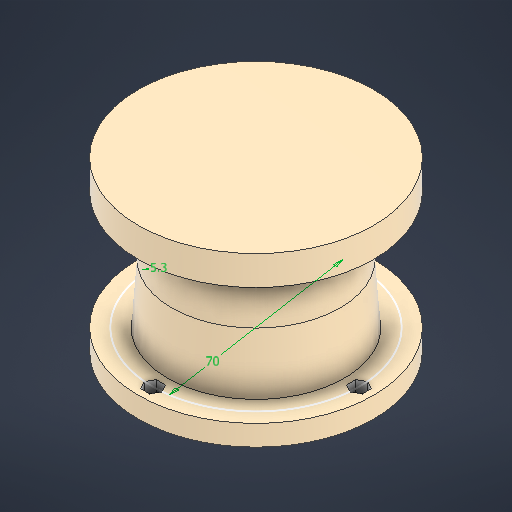
# Autodesk Inventor part: spool
Saved by Autodesk Inventor 2026.2 (Build 302298010, 298A)
## iProperties
Created: 2026-02-24
Part Number: spool
Material: ABS Plastic
Document SubType Name: Modeling
Designer: Luke
Density: 1.06 g/cm^3
Appearance: Smooth - White
Author: Luke
Autodesk Inventor part; units mm, degrees
ref_plane "YZ Plane" through (0, 0, 0) normal (1, 0, 0) x (0, 1, 0)
ref_plane "XZ Plane" through (0, 0, 0) normal (0, 1, 0) x (-1, 0, 0)
ref_plane "XY Plane" through (0, 0, 0) normal (0, 0, 1) x (1, 0, 0)
sketch "Sketch1" plane through (0, 0, 0) normal (0, 1, 0) x (-1, 0, 0)
  circle A0 centre (0, 0) radius 30
  circle A1 centre (0, 0) radius 45
  circle A2 centre (0, 0) radius 20
  dimension "d0" = 60
  dimension "d1" = 90
  dimension "d2" = 40
  constraints: 3 centre point, 3 coincident
  measures "d0" diameter of A0
  measures "d1" diameter of A1
  measures "d2" diameter of A2
extrude "Extrusion1" add sketch "Sketch1" along normal blind 20 draft -4 contours A0
sketch "Sketch2" plane through (0, 20, 0) normal (0, 1, 0) x (1, 0, 0)
  circle A0 centre (0, 0) radius 28.6015
  circle A1 centre (0, 0) radius 21.3985
  constraints: 2 centre point, 2 coincident
extrude "Extrusion2" add sketch "Sketch2" along normal blind 20 draft 4
sketch "Sketch3" plane through (0, 40, 0) normal (0, 1, 0) x (1, 0, 0)
  circle A0 centre (0, 0) radius 40
  dimension "d7" = 80
  constraints: 1 centre point, 1 coincident
  measures "d7" diameter of A0
extrude "Extrusion3" add sketch "Sketch3" along normal blind 10
sketch "Sketch4" plane through (0, 0, 0) normal (0, -1, 0) x (1, 0, 0)
  circle A0 centre (0, 0) radius 40
  dimension "d10" = 80
  constraints: 1 centre point, 1 coincident
  measures "d10" diameter of A0
extrude "Extrusion4" add sketch "Sketch4" along normal blind 10
ref_plane "Work Plane1" through (0, -8, 0) normal (0, -1, 0) x (1, 0, 0)
sketch "Sketch7" plane through (0, -10, 0) normal (0, -1, 0) x (1, 0, 0)
  circle A0 centre (0, 0) radius 40
  constraints: 1 centre point, 1 coincident
extrude "Extrusion12" cut sketch "Sketch7" against normal blind 3
sketch "Sketch8" plane through (0, -7, 0) normal (0, -1, 0) x (1, 0, 0)
  circle A0 centre (0, 0) radius 25
  dimension "d42" = 50
  constraints: 1 centre point, 1 coincident
  measures "d42" diameter of A0
extrude "Extrusion13" cut sketch "Sketch8" against normal blind 5
sketch "Sketch9" plane through (0, 0, 0) normal (0, 1, 0) x (1, 0, 0)
  circle A0 centre (0, 0) radius 35
  line L0 (-37.65, 1.53) -> (-35, 3.06)
  line L1 (-35, 3.06) -> (-32.35, 1.53)
  line L2 (-32.35, 1.53) -> (-32.35, -1.53)
  line L3 (-32.35, -1.53) -> (-35, -3.06)
  line L4 (-35, -3.06) -> (-37.65, -1.53)
  line L5 (-37.65, -1.53) -> (-37.65, 1.53)
  line L6 (0, 0) -> (-35, 0) construction
  circle A1 centre (-35, 0) radius 2.65
  point P0 (-33.675, 2.295)
  point P1 (-36.325, -2.295)
  dimension "d45" = 70
  dimension "d46" = 5.3
  constraints: 14 end point, 2 coincident, 2 midpoint, 1 centre point, 1 horizontal, 1 horizontal alignment, 1 vertical, 15 other
  measures "d46" distance of point (-33.675, 2.295) point (-36.325, -2.295)
extrude "Extrusion14" cut sketch "Sketch9" against normal through all contours L1 A1 A0 | A0 A1 L0 L1 | L3 L4 A1 A0 | A0 A1 L3 | A1 A0 | A0 A1 | L1 L2 A1 | A1 L2 L3 | A1 L5 L0 | L4 L5 A1
pattern_circular "Circular Pattern1" count 4 over 360 about axis through (0, 0, 0) along (0, -1, 0) of "Extrusion14"
sketch "Sketch10" plane through (0, 0, 0) normal (0, 0, 1) x (1, 0, 0)
  point P0 (0, 0)
sketch "Sketch11" plane through (0, 0, 0) normal (0, 0, 1) x (1, 0, 0)
  line L0 (-24.5677, 41.8645) -> (0, 41.8645)
  line L1 (0, 41.8645) -> (0, 0)
  line L2 (0, 0) -> (-24.5677, 0)
  line L3 (-24.5677, 0) -> (-24.5677, 41.8645)
  constraints: 8 end point, 2 parallel, 1 horizontal, 1 perpendicular
revolve "Revolution1" add sketch "Sketch11" angle 360 about axis through (0, 41.8645, 0) along (0, -1, 0)
sketch "Sketch12" plane through (0, -7, 0) normal (0, -1, 0) x (1, 0, 0)
  point P0 (0, 0)
sketch "Sketch13" plane through (0, -7, 0) normal (0, -1, 0) x (1, 0, 0)
  line L0 (0, 35) -> (0, 0) construction
  circle A0 centre (0, 35) radius 3.15
  circle A1 centre (0, 35) radius 1.25
  dimension "d53" = 35
  dimension "d54" = 6.3
  dimension "d57" = 2.5
  constraints: 2 centre point, 2 coincident, 2 end point, 1 vertical
  measures "d53" distance of L0.start L0.end
  measures "d54" diameter of A0
  measures "d57" diameter of A1
extrude "Extrusion15" add sketch "Sketch13" against normal blind 2
pattern_circular "Circular Pattern2" count 4 over 360 about axis through (0, 0, 0) along (0, -1, 0) of "Extrusion15"
body "Solid1"
